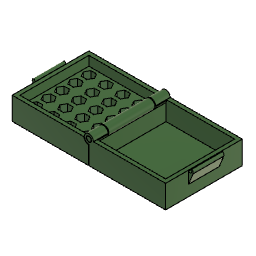
Lab03 v5 (Autodesk Fusion 360 design; units mm, degrees)
Autodesk Fusion 360 part; units mm, degrees
note: some values were not read from the file. Set by a fixed rule: which face or edge a step refers to.
sketch "Sketch1" plane through (0, 0, 0) normal (0, 1, 0) x (1, 0, 0)
  line L0 (0, 0) -> (50, 0)
  line L1 (0, 0) -> (-50, 0)
  line L2 (0, 0) -> (0, 15)
  line L3 (0, 15) -> (-50, 15)
  line L4 (-50, 15) -> (-50, 0)
  line L5 (0, 15) -> (50, 15)
  line L6 (50, 15) -> (50, 0)
  circle A0 centre (0, 0) radius 1.5
  circle A1 centre (0, 0) radius 1.75
  circle A2 centre (0, 0) radius 3
  circle A3 centre (0, 0) radius 3.25
  dimension "d1" = 50
  dimension "d2" = 50
  dimension "d3" = 15
  dimension "d4" = 50
  dimension "d5" = 50
  dimension "d6" = 3
  dimension "d7" = 3.5
  dimension "d8" = 6
  dimension "d9" = 6.5
  constraint coincident L0.start L1.start
  constraint horizontal L0
  constraint parallel L0 L1
  constraint perpendicular L1 L2
  constraint perpendicular L2 L3
  constraint perpendicular L2 L5
  constraint concentric A0 A2
  measures "d1" distance of L0.start L0.end
  measures "d2" distance of L0.start L1.end
  measures "d3" distance of L0.start L2.end
  measures "d4" distance of L2.end L3.end
  measures "d5" distance of L2.end L5.end
  measures "d6" diameter of A0
  measures "d7" diameter of A1
  measures "d8" diameter of A2
  measures "d9" diameter of A3
extrude "Extrude1" add sketch "Sketch1" along normal blind 50 contours L0 L2 A0 | L0 L2 A0 A1 | L0 L2 A1 A2 | L0 L2 A2 A3 | L0 L2 L5 L6 A3 makes body 1
extrude "Extrude2" add sketch "Sketch1" along normal blind 50 separate body contours L1 L2 A0 | L1 L2 A0 A1 | L1 L2 A1 A2 | L1 L2 A2 A3 | L1 L2 L3 L4 A3 makes body 2
move_face "OffsetFaces1" offset -0.25 5 faces at (0, 16.6667, -0.5) (0, 33.3333, -1.5833) (0, 16.6667, -2.1667) (0, 16.6667, -3.0833) (0, 16.6667, -7.1667) on bodies 2
move_face "OffsetFaces2" offset -0.25 5 faces at (-0.6667, 16.6667, 0) (-1.5833, 33.3333, 0) (-2.1667, 16.6667, 0) (-3.0833, 16.6667, 0) (-34.4167, 33.3333, 0) on bodies 2
move_face "OffsetFaces3" offset -0.25 5 faces at (0.5, 16.6667, 0) (1.5833, 16.6667, 0) (2.1667, 16.6667, 0) (3.0833, 16.6667, 0) (18.8333, 16.6667, 0) on bodies 1
move_face "OffsetFaces4" offset -0.25 5 faces at (0, 16.6667, -0.6667) (0, 33.3333, -1.5833) (0, 16.6667, -2.1667) (0, 16.6667, -3.0833) (0, 16.6667, -7.1667) on bodies 1
shell "Shell1" thickness 2.5 removed faces 10 at (0.6667, 16.6667, -0.25) at (1.5833, 16.6667, -0.25) at (18.8333, 16.6667, -0.25) at (3.0833, 16.6667, -0.25) at (2.1667, 16.6667, -0.25) at (-0.6667, 16.6667, -0.25) at (-1.5833, 33.3333, -0.25) at (-2.1667, 16.6667, -0.25) at (-3.0833, 16.6667, -0.25) at (-18.8333, 16.6667, -0.25) on bodies 1 2
extrude "Extrude3" cut sketch "Sketch1" along normal blind 50 contours L0 L2 A0 | L0 L1 A0 | L1 L2 A0 | L0 L2 A0 A1 | L0 L1 A0 A1 | L1 L2 A0 A1 | L0 L2 A1 A2 | L0 L1 A1 A2 | L1 L2 A1 A2 | L0 L2 A2 A3 | L0 L1 A2 A3 | L1 L2 A2 A3 bodies 1 2
extrude "Extrude4" add sketch "Sketch1" along normal blind 40 contours L0 L2 A0 A1 | L0 L1 A0 A1 | L1 L2 A0 A1 | L0 L2 A1 A2 | L0 L1 A1 A2 | L1 L2 A1 A2 | L1 L2 A2 A3 bodies 2
extrude "Extrude5" add sketch "Sketch1" along normal blind 50 contours L0 L2 A0 | L0 L1 A0 | L1 L2 A0 bodies 2
extrude "Extrude6" cut sketch "Sketch1" along normal blind 10 contours L0 L2 A0 A1 | L0 L1 A0 A1 | L1 L2 A0 A1 | L0 L2 A1 A2 | L0 L1 A1 A2 | L1 L2 A1 A2 | L1 L2 A2 A3 bodies 2
extrude "Extrude7" add sketch "Sketch1" along normal blind 50 contours L0 L2 A1 A2 | L0 L1 A1 A2 | L1 L2 A1 A2 | L0 L2 A2 A3 bodies 1
extrude "Extrude8" cut sketch "Sketch1" along normal blind 40.5 contours L0 L2 A1 A2 | L0 L1 A1 A2 | L1 L2 A1 A2 | L0 L2 A2 A3 bodies 1
extrude "Extrude9" add sketch "Sketch1" along normal blind 9.5 contours L0 L2 A1 A2 | L0 L1 A1 A2 | L1 L2 A1 A2 | L0 L2 A2 A3 bodies 1
copy_body "Body->Comp1" bodies 1 removing the originals makes body 3 in component "top"
copy_body "Body->Comp2" bodies 2 removing the originals makes body 4 in component "bottom"
move_face "OffsetFaces1'" offset 0.25 1 faces at (49.1667, 17.5, -0.25) on bodies 3 in component "top"
fillet "Fillet1" radius 0.25 1 edges at (3.25, 44, 0) on bodies 3 in component "top"
fillet "Fillet2" radius 0.25 1 edges at (3.25, 6, 0) on bodies 3 in component "top"
fillet "Fillet1'" radius 0.25 1 edges at (-3.25, 25, 0) on bodies 4 in component "bottom"
fillet "Fillet2'" radius 0.25 1 edges at (0, 25, -3.25) on bodies 4 in component "bottom"
move_face "OffsetFaces2'" offset 0.24 1 faces at (0.25, 30.1667, -11.0801) on bodies 3 in component "top"
fillet "Fillet3" radius 0.1 1 edges at (0, 4.75, -3.25) on bodies 3 in component "top"
fillet "Fillet4" radius 0.1 1 edges at (0, 45.25, -3.25) on bodies 3 in component "top"
extrude "Extrude1'" add 1 faces at (-17.6667, 32.5, -12.5) along direction (0, 0, 1) blind 6.125 on bodies 4 bodies 4 in component "bottom"
sketch "Sketch2" plane through (0, 0, -6.375) normal (0, 0, 1) x (-1, 0, 0)
  line L0 (47.5, -2.5) -> (2.75, -2.5)
  line L1 (2.75, -2.5) -> (2.75, -47.5)
  line L2 (2.75, -47.5) -> (47.5, -47.5)
  line L3 (47.5, -47.5) -> (47.5, -2.5)
  line L4 (47.5, -47.5) -> (42.5, -47.5)
  line L5 (42.5, -47.5) -> (42.5, -42.5)
  line L6 (44.3187, -45.65) -> (46.1373, -42.5)
  line L7 (46.1373, -42.5) -> (44.3187, -39.35)
  line L8 (44.3187, -39.35) -> (40.6813, -39.35)
  line L9 (40.6813, -39.35) -> (38.8627, -42.5)
  line L10 (38.8627, -42.5) -> (40.6813, -45.65)
  line L11 (40.6813, -45.65) -> (44.3187, -45.65)
  line L12 (33.3187, -39.35) -> (29.6813, -39.35)
  line L13 (35.1373, -42.5) -> (33.3187, -39.35)
  line L14 (33.3187, -45.65) -> (35.1373, -42.5)
  line L15 (29.6813, -45.65) -> (33.3187, -45.65)
  line L16 (27.8627, -42.5) -> (29.6813, -45.65)
  line L17 (29.6813, -39.35) -> (27.8627, -42.5)
  line L18 (22.3187, -39.35) -> (18.6813, -39.35)
  line L19 (24.1373, -42.5) -> (22.3187, -39.35)
  line L20 (22.3187, -45.65) -> (24.1373, -42.5)
  line L21 (18.6813, -45.65) -> (22.3187, -45.65)
  line L22 (16.8627, -42.5) -> (18.6813, -45.65)
  line L23 (18.6813, -39.35) -> (16.8627, -42.5)
  line L24 (11.3187, -39.35) -> (7.6813, -39.35)
  line L25 (13.1373, -42.5) -> (11.3187, -39.35)
  line L26 (11.3187, -45.65) -> (13.1373, -42.5)
  line L27 (7.6813, -45.65) -> (11.3187, -45.65)
  line L28 (5.8627, -42.5) -> (7.6813, -45.65)
  line L29 (7.6813, -39.35) -> (5.8627, -42.5)
  line L30 (44.3187, -30.6) -> (40.6813, -30.6)
  line L31 (46.1373, -33.75) -> (44.3187, -30.6)
  line L32 (44.3187, -36.9) -> (46.1373, -33.75)
  line L33 (40.6813, -36.9) -> (44.3187, -36.9)
  line L34 (38.8627, -33.75) -> (40.6813, -36.9)
  line L35 (40.6813, -30.6) -> (38.8627, -33.75)
  line L36 (33.3187, -30.6) -> (29.6813, -30.6)
  line L37 (35.1373, -33.75) -> (33.3187, -30.6)
  line L38 (33.3187, -36.9) -> (35.1373, -33.75)
  line L39 (29.6813, -36.9) -> (33.3187, -36.9)
  line L40 (27.8627, -33.75) -> (29.6813, -36.9)
  line L41 (29.6813, -30.6) -> (27.8627, -33.75)
  line L42 (22.3187, -30.6) -> (18.6813, -30.6)
  line L43 (24.1373, -33.75) -> (22.3187, -30.6)
  line L44 (22.3187, -36.9) -> (24.1373, -33.75)
  line L45 (18.6813, -36.9) -> (22.3187, -36.9)
  line L46 (16.8627, -33.75) -> (18.6813, -36.9)
  line L47 (18.6813, -30.6) -> (16.8627, -33.75)
  line L48 (11.3187, -30.6) -> (7.6813, -30.6)
  line L49 (13.1373, -33.75) -> (11.3187, -30.6)
  line L50 (11.3187, -36.9) -> (13.1373, -33.75)
  line L51 (7.6813, -36.9) -> (11.3187, -36.9)
  line L52 (5.8627, -33.75) -> (7.6813, -36.9)
  line L53 (7.6813, -30.6) -> (5.8627, -33.75)
  line L54 (44.3187, -21.85) -> (40.6813, -21.85)
  line L55 (46.1373, -25) -> (44.3187, -21.85)
  line L56 (44.3187, -28.15) -> (46.1373, -25)
  line L57 (40.6813, -28.15) -> (44.3187, -28.15)
  line L58 (38.8627, -25) -> (40.6813, -28.15)
  line L59 (40.6813, -21.85) -> (38.8627, -25)
  line L60 (33.3187, -21.85) -> (29.6813, -21.85)
  line L61 (35.1373, -25) -> (33.3187, -21.85)
  line L62 (33.3187, -28.15) -> (35.1373, -25)
  line L63 (29.6813, -28.15) -> (33.3187, -28.15)
  line L64 (27.8627, -25) -> (29.6813, -28.15)
  line L65 (29.6813, -21.85) -> (27.8627, -25)
  line L66 (22.3187, -21.85) -> (18.6813, -21.85)
  line L67 (24.1373, -25) -> (22.3187, -21.85)
  line L68 (22.3187, -28.15) -> (24.1373, -25)
  line L69 (18.6813, -28.15) -> (22.3187, -28.15)
  line L70 (16.8627, -25) -> (18.6813, -28.15)
  line L71 (18.6813, -21.85) -> (16.8627, -25)
  line L72 (11.3187, -21.85) -> (7.6813, -21.85)
  line L73 (13.1373, -25) -> (11.3187, -21.85)
  line L74 (11.3187, -28.15) -> (13.1373, -25)
  line L75 (7.6813, -28.15) -> (11.3187, -28.15)
  line L76 (5.8627, -25) -> (7.6813, -28.15)
  line L77 (7.6813, -21.85) -> (5.8627, -25)
  line L78 (44.3187, -13.1) -> (40.6813, -13.1)
  line L79 (46.1373, -16.25) -> (44.3187, -13.1)
  line L80 (44.3187, -19.4) -> (46.1373, -16.25)
  line L81 (40.6813, -19.4) -> (44.3187, -19.4)
  line L82 (38.8627, -16.25) -> (40.6813, -19.4)
  line L83 (40.6813, -13.1) -> (38.8627, -16.25)
  line L84 (33.3187, -13.1) -> (29.6813, -13.1)
  line L85 (35.1373, -16.25) -> (33.3187, -13.1)
  line L86 (33.3187, -19.4) -> (35.1373, -16.25)
  line L87 (29.6813, -19.4) -> (33.3187, -19.4)
  line L88 (27.8627, -16.25) -> (29.6813, -19.4)
  line L89 (29.6813, -13.1) -> (27.8627, -16.25)
  line L90 (22.3187, -13.1) -> (18.6813, -13.1)
  line L91 (24.1373, -16.25) -> (22.3187, -13.1)
  line L92 (22.3187, -19.4) -> (24.1373, -16.25)
  line L93 (18.6813, -19.4) -> (22.3187, -19.4)
  line L94 (16.8627, -16.25) -> (18.6813, -19.4)
  line L95 (18.6813, -13.1) -> (16.8627, -16.25)
  line L96 (11.3187, -13.1) -> (7.6813, -13.1)
  line L97 (13.1373, -16.25) -> (11.3187, -13.1)
  line L98 (11.3187, -19.4) -> (13.1373, -16.25)
  line L99 (7.6813, -19.4) -> (11.3187, -19.4)
  line L100 (5.8627, -16.25) -> (7.6813, -19.4)
  line L101 (7.6813, -13.1) -> (5.8627, -16.25)
  line L102 (44.3187, -4.35) -> (40.6813, -4.35)
  line L103 (46.1373, -7.5) -> (44.3187, -4.35)
  line L104 (44.3187, -10.65) -> (46.1373, -7.5)
  line L105 (40.6813, -10.65) -> (44.3187, -10.65)
  line L106 (38.8627, -7.5) -> (40.6813, -10.65)
  line L107 (40.6813, -4.35) -> (38.8627, -7.5)
  line L108 (33.3187, -4.35) -> (29.6813, -4.35)
  line L109 (35.1373, -7.5) -> (33.3187, -4.35)
  line L110 (33.3187, -10.65) -> (35.1373, -7.5)
  line L111 (29.6813, -10.65) -> (33.3187, -10.65)
  line L112 (27.8627, -7.5) -> (29.6813, -10.65)
  line L113 (29.6813, -4.35) -> (27.8627, -7.5)
  line L114 (22.3187, -4.35) -> (18.6813, -4.35)
  line L115 (24.1373, -7.5) -> (22.3187, -4.35)
  line L116 (22.3187, -10.65) -> (24.1373, -7.5)
  line L117 (18.6813, -10.65) -> (22.3187, -10.65)
  line L118 (16.8627, -7.5) -> (18.6813, -10.65)
  line L119 (18.6813, -4.35) -> (16.8627, -7.5)
  line L120 (11.3187, -4.35) -> (7.6813, -4.35)
  line L121 (13.1373, -7.5) -> (11.3187, -4.35)
  line L122 (11.3187, -10.65) -> (13.1373, -7.5)
  line L123 (7.6813, -10.65) -> (11.3187, -10.65)
  line L124 (5.8627, -7.5) -> (7.6813, -10.65)
  line L125 (7.6813, -4.35) -> (5.8627, -7.5)
  point P0 (42.5, -42.5)
  dimension "d55" = 5
  dimension "d56" = 5
  dimension "d57" = 3.15
  dimension "d60" = -33
  dimension "d61" = 35
  constraint coincident L2.end L3.start
  constraint perpendicular L3 L4
  constraint perpendicular L4 L5
  constraint coincident P0 L5.end
  measures "d55" distance of L2.end L4.end
  measures "d56" distance of L4.end P0
  measures "d57" distance of P0 L11
extrude "Extrude2'" cut sketch "Sketch2" against normal blind 6.25 contours L6 L7 L8 L9 L10 L11 | L12 L13 L14 L15 L16 L17 | L18 L19 L20 L21 L22 L23 | L24 L25 L26 L27 L28 L29 | L30 L31 L32 L33 L34 L35 | L36 L37 L38 L39 L40 L41 | L42 L43 L44 L45 L46 L47 | L48 L49 L50 L51 L52 L53 | L54 L55 L56 L57 L58 L59 | L60 L61 L62 L63 L64 L65 | L66 L67 L68 L69 L70 L71 | L72 L73 L74 L75 L76 L77 | L78 L79 L80 L81 L82 L83 | L84 L85 L86 L87 L88 L89 | L90 L91 L92 L93 L94 L95 | L96 L97 L98 L99 L100 L101 | L102 L103 L104 L105 L106 L107 | L108 L109 L110 L111 L112 L113 | L114 L115 L116 L117 L118 L119 | L120 L121 L122 L123 L124 L125 bodies 4 in component "bottom"
sketch "Sketch3" plane through (0, 0, 0) normal (0, -1, 0) x (1, 0, 0)
  arc A0 (0, 3.2064) -> (-0.01, 3.25) centre (-0.1, 3.2064) ccw
  line L0 (-0.01, 3.25) -> (-0.01, 15)
  line L1 (-0.01, 15) -> (-50, 15)
  line L2 (-50, 15) -> (-50, 0)
  line L3 (-50, 0) -> (-3, 0)
  arc A1 (-3, 0) -> (0, 3) centre (0, 0) ccw
  line L4 (0, 3) -> (0, 3.2064)
  circle A2 centre (0, 0) radius 1.75
  line L5 (-50, 0) -> (-50, 8)
  line L6 (-50, 0) -> (-50, -8)
  line L7 (-50, 0) -> (-51, 0)
  circle A3 centre (-51, 0) radius 0.95
  circle A4 centre (-51, 0) radius 0.8
  circle A5 centre (-51, 0) radius 1.1
  line L8 (-50, -8) -> (-51.7801, -0.1775)
  circle A6 centre (-51, 0) radius 2
  line L9 (-50, 8) -> (-52.861, 0.7326)
  dimension "d65" = 8
  dimension "d66" = 8
  dimension "d67" = 1
  dimension "d68" = 1.9
  dimension "d69" = 1.6
  dimension "d70" = 2.2
  dimension "d71" = 4
  constraint coincident L2.end L3.start
  constraint perpendicular L3 L5
  constraint perpendicular L3 L6
  constraint perpendicular L6 L7
  constraint coincident L7.end A3.centre
  constraint concentric A4 A5
  constraint coincident A4 L8.end
  constraint tangent A4 L8
  constraint concentric A3 A6
  constraint coincident A6 L9.end
  constraint tangent A6 L9
  measures "d65" distance of L2.end L5.end
  measures "d66" distance of L2.end L6.end
  measures "d67" distance of L2.end L7.end
  measures "d68" diameter of A3
  measures "d69" diameter of A4
  measures "d70" diameter of A5
  measures "d71" diameter of A6
extrude "Extrude1''" add sketch "Sketch3" against normal blind 35 contours L2 L5 A6 L9 | L2 L5 A5 L8 A6 sketch seen with x (-1, 0, 0) y (0, 1, 0) z (0, 0, -1) at (0, 0, 0) bodies 3 in component "top"
extrude "Extrude2''" cut sketch "Sketch3" against normal blind 15 contours L2 L5 A6 L9 | L2 L5 A5 L8 A6 sketch seen with x (-1, 0, 0) y (0, 1, 0) z (0, 0, -1) at (0, 0, 0) bodies 3 in component "top"
extrude "Extrude3'" add sketch "Sketch3" against normal blind 35 contours L6 A5 L8 A6 | L6 L8 A6 | L6 L7 A3 A5 L8 | L7 A3 A4 L8 | L7 A3 A4 L8 | A4 bodies 4 in component "bottom"
extrude "Extrude4'" cut sketch "Sketch3" against normal blind 15 contours L6 A5 L8 A6 | L6 L8 A6 | L6 L7 A3 A5 L8 | L7 A3 A4 L8 | L7 A3 A4 L8 | A4 bodies 4 in component "bottom"
fillet "Fillet3'" radius 2.05 1 edges at (-50, 25, 0) on bodies 4 in component "bottom"
fillet "Fillet5" radius 0.4 1 edges at (51.3733, 25, 1.9648) on bodies 3 in component "top"
move_face "OffsetFaces3'" offset -0.01 1 faces at (50.9903, 28.3333, -1.1) on bodies 3 in component "top"
move_face "OffsetFaces1''" offset 0.05 1 faces at (-50.9385, 28.3333, 0.948) on bodies 4 in component "bottom"
component "top" placed x (-1, 0, 0) y (0, 1, 0) z (0, 0, -1) at (0, 0, 0)
component "bottom" placed x (1, 0, 0) y (0, 1, 0) z (0, 0, 1) at (0, 0, 0)
equation "d31 = 1 mm + 8.50 mm"
equation "d53 = ( ( 12.25 / 2 ) * 1 mm )"
equation "d57 = ( 6.3 / 2 ) * 1 mm"
equation "d62 = -( ( 12.5 / 2 ) * 1 mm )"
named bodies: "top", "bottom"
